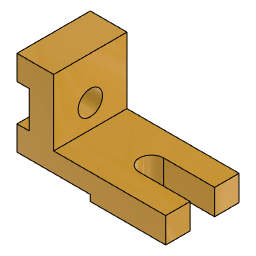
Exercise-2 v1 (Autodesk Fusion 360 design; units mm, degrees)
Autodesk Fusion 360 part; units mm, degrees
sketch "Sketch1" plane through (0, 0, 0) normal (0, 0, 1) x (1, 0, 0)
  line L0 (73, -36) -> (-73, -36)
  line L1 (-73, -36) -> (-73, 36)
  line L2 (-73, 36) -> (73, 36)
  line L3 (73, 36) -> (73, -36)
  line L4 (73, -36) -> (-73, 36) construction
  line L5 (-73, -36) -> (73, 36) construction
  line L6 (-73, -36) -> (-1, -36)
  line L7 (-1, -36) -> (-1, 14)
  line L8 (-1, 14) -> (-73, 14)
  line L9 (-73, 14) -> (-73, -36)
  line L10 (23, 12) -> (73, 12)
  line L11 (23, -12) -> (73, -12)
  arc A0 (24.2094, 11.9389) -> (24.2094, -11.9389) centre (23, 0) ccw
  dimension "d1" = 146
  dimension "d2" = 72
  dimension "d3" = 72
  dimension "d4" = 50
  dimension "d5" = 24
  dimension "d6" = 50
  constraint horizontal L0
  constraint perpendicular L0 L1
  constraint parallel L0 L2
  constraint parallel L1 L3
  constraint coincident L4 origin
  constraint coincident L5 origin
  constraint horizontal L6
  constraint vertical L7
  constraint horizontal L8
  constraint vertical L9
  constraint coincident L10.start A0
  constraint coincident L3 L10.end
  constraint perpendicular L3 L10
  constraint coincident L11.start A0
  constraint coincident L3 L11.end
  constraint tangent L11 A0
  constraint tangent L10 A0
  constraint coincident L4 A0.end
  constraint coincident L5 A0.start
  measures "d1" distance of L1.end L2.end
  measures "d2" distance of L0.end L1.end
  measures "d3" distance of L0.end L6.end
  measures "d4" distance of L0.end L8.end
  measures "d5" diameter of A0
  measures "d6" distance of L3 A0.centre
extrude "Extrude1" add sketch "Sketch1" along normal blind 25 contours L0 L1 L2 L3 L7 L8 L10 L11 A0 | L0 L1 L6 L7 L8 L9
extrude "Extrude2" cut sketch "Sketch1" along normal blind 6 contours L0 L1 L6 L7 L8 L9
sketch "Sketch2" plane through (0, 0, 25) normal (0, 0, 1) x (-1, 0, 0)
  arc A0 (-23, -12) -> (-23, 12) centre (-23, 0) ccw
  line L0 (-23, -12) -> (-73, -12)
  line L1 (-73, -12) -> (-73, -36)
  line L2 (-73, -36) -> (73, -36)
  line L3 (73, -36) -> (73, 36)
  line L4 (73, 36) -> (-73, 36)
  line L5 (-73, 36) -> (-73, 12)
  line L6 (-73, 12) -> (-23, 12)
  line L7 (73, 36) -> (37, 36)
  line L8 (37, 36) -> (37, -36)
  line L9 (37, -36) -> (73, -36)
  line L10 (73, -36) -> (73, 36)
  dimension "d11" = 36
  dimension "d12" = 72
  constraint horizontal L7
  constraint vertical L8
  constraint horizontal L9
  constraint vertical L10
  constraint coincident L3.end L4.start
  measures "d11" distance of L3.end L7.end
  measures "d12" distance of L3.end L2.end
extrude "Extrude3" add sketch "Sketch2" along normal blind 65 contours L2 L3 L4 L7 L8 L9 L10
sketch "Sketch3" plane through (-73, 0, 0) normal (-1, 0, 0) x (0, -1, 0)
  line L0 (-14, 0) -> (-14, 6)
  line L1 (-14, 6) -> (36, 6)
  line L2 (36, 6) -> (36, 90)
  line L3 (36, 90) -> (-36, 90)
  line L4 (-36, 90) -> (-36, 0)
  line L5 (-36, 0) -> (-14, 0)
  circle A0 centre (0, 48) radius 12
  circle A1 centre (0, 48) radius 30
  line L6 (-36, 90) -> (36, 90)
  line L7 (36, 90) -> (36, 66)
  line L8 (36, 66) -> (-36, 66)
  line L9 (-36, 66) -> (-36, 90)
  line L10 (36, 6) -> (-36.1808, 6)
  line L11 (-36.1808, 6) -> (-36.1808, 30)
  line L12 (-36.1808, 30) -> (36, 30)
  line L13 (36, 30) -> (36, 6)
  dimension "d15" = 24
  dimension "d16" = 60
  dimension "d17" = 48
  dimension "d18" = 24
  dimension "d19" = 24
  constraint concentric A0 A1
  constraint horizontal L6
  constraint vertical L7
  constraint horizontal L8
  constraint vertical L9
  constraint coincident L2 L7.end
  constraint coincident L3.end L4.start
  constraint horizontal L10
  constraint vertical L11
  constraint horizontal L12
  constraint vertical L13
  constraint coincident L1.end L2.start
  measures "d15" diameter of A0
  measures "d16" diameter of A1
  measures "d17" distance of L5 A0.centre
  measures "d18" distance of L2.end L7.end
  measures "d19" distance of L1.end L12.end
extrude "Extrude4" cut sketch "Sketch3" against normal blind 36 contours A0
extrude "Extrude5" cut sketch "Sketch3" against normal blind 12 contours L2 A1 L8 L12 | L4 A1 L8 L12 | A1 L8 L12 | A1 L12 | A1 L8
